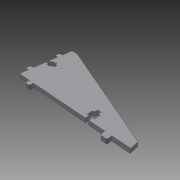
# Autodesk Inventor part: wiring_brace
Saved by Autodesk Inventor 2014 (Build 180170000, 170)
## iProperties
Created: 2013-12-07
Part Number: wiring_brace
Material: Generic
Document SubType Name: Modeling
Designer: buben
Density: 1 g/cm^3
Appearance: Default
Author: buben
Subject: Laser Cutted
Autodesk Inventor part; units mm, degrees
ref_plane "YZ Plane" through (0, 0, 0) normal (1, 0, 0) x (0, 1, 0)
ref_plane "XZ Plane" through (0, 0, 0) normal (0, 1, 0) x (-1, 0, 0)
ref_plane "XY Plane" through (0, 0, 0) normal (0, 0, 1) x (1, 0, 0)
sketch "Sketch1" plane through (0, 0, 0) normal (0, 0, 1) x (1, 0, 0)
  line L0 (0, 81) -> (0, 0)
  line L1 (0, 0) -> (161.5, 0)
  line L2 (161.5, 0) -> (161.5, 10)
  line L3 (161.5, 10) -> (10, 81)
  line L4 (10, 81) -> (0, 81)
  dimension "d0" = 161.5
  dimension "d1" = 81
  dimension "d2" = 10
  dimension "d3" = 10
  constraints: 10 end point, 2 parallel, 1 perpendicular, 1 vertical
  measures "d0" distance of L0.end L1.end
  measures "d1" distance of L0.start L0.end
  measures "d2" distance of L3.end L0.start
  measures "d3" distance of L1.end L2.end
extrude "Extrusion1" add sketch "Sketch1" along normal blind 6
sketch "Sketch2" plane through (0, 0, 6) normal (0, 0, 1) x (1, 0, 0)
  line L0 (0, 81) -> (0, 0) projected
  line L1 (0, 0) -> (161.5, 0) projected
  line L2 (161.5, 0) -> (161.5, 10) projected
  line L3 (16.3, 42.75) -> (16.3, 38.25)
  line L4 (0, 38.25) -> (0, 42.75)
  line L5 (5, 45.25) -> (12.3, 45.25)
  line L6 (12.3, 35.75) -> (5, 35.75)
  line L7 (0, 42.75) -> (5, 42.75)
  line L8 (12.3, 42.75) -> (16.3, 42.75)
  line L9 (16.3, 38.25) -> (12.3, 38.25)
  line L10 (5, 38.25) -> (0, 38.25)
  line L11 (5, 35.75) -> (5, 38.25)
  line L12 (5, 42.75) -> (5, 45.25)
  line L13 (12.3, 45.25) -> (12.3, 42.75)
  line L14 (12.3, 38.25) -> (12.3, 35.75)
  line L15 (109.25, 16.3) -> (113.75, 16.3)
  line L16 (113.75, 0) -> (109.25, 0)
  line L17 (116.25, 12.3) -> (116.25, 5)
  line L18 (106.75, 5) -> (106.75, 12.3)
  line L19 (106.75, 12.3) -> (109.25, 12.3)
  line L20 (113.75, 12.3) -> (116.25, 12.3)
  line L21 (116.25, 5) -> (113.75, 5)
  line L22 (109.25, 5) -> (106.75, 5)
  line L23 (109.25, 0) -> (109.25, 5)
  line L24 (109.25, 12.3) -> (109.25, 16.3)
  line L25 (113.75, 16.3) -> (113.75, 12.3)
  line L26 (113.75, 5) -> (113.75, 0)
  point P0 (16.3, 40.5)
  point P1 (0, 40.5)
  point P2 (111.5, 16.3)
  dimension "d6" = 4.5
  dimension "d7" = 2.5
  dimension "d8" = 2.5
  dimension "d9" = 5
  dimension "d10" = 7.3
  dimension "d11" = 4
  dimension "d12" = 4.5
  dimension "d13" = 5
  dimension "d14" = 7.3
  dimension "d15" = 4
  dimension "d16" = 2.5
  dimension "d17" = 2.5
  dimension "d18" = 50
  constraints: 48 end point, 20 parallel, 10 collinear, 8 perpendicular, 6 horizontal, 3 midpoint, 1 horizontal alignment
  measures "d6" distance of L3.start L3.end
  measures "d7" distance of L5.end L8.start
  measures "d8" distance of L9.end L6.start
  measures "d9" distance of L10.start L4.start
  measures "d10" distance of L6.start L6.end
  measures "d11" distance of L3.end L9.end
  measures "d12" distance of L15.start L15.end
  measures "d13" distance of L16.end L22.start
  measures "d14" distance of L18.start L18.end
  measures "d15" distance of L19.end L15.start
  measures "d16" distance of L18.end L19.end
  measures "d17" distance of L20.start L17.start
  measures "d18" distance from line of L2 point (111.5, 16.3)
extrude "Extrusion2" cut sketch "Sketch2" against normal blind 6
sketch "Sketch3" plane through (0, 0, 6) normal (0, 0, 1) x (1, 0, 0)
  line L0 (0, 38.25) -> (0, 0) projected
  line L1 (0, 0) -> (109.25, 0) projected
  line L2 (113.75, 0) -> (161.5, 0) projected
  line L3 (10, 81) -> (0, 81) projected
  line L4 (0, 81) -> (0, 42.75) projected
  line L5 (0, 65) -> (-4, 65)
  line L6 (-6, 63) -> (-6, 59)
  line L7 (-4, 57) -> (0, 57)
  line L8 (0, 57) -> (0, 65)
  line L9 (0, 20) -> (-4, 20)
  line L10 (-6, 18) -> (-6, 14)
  line L11 (-4, 12) -> (0, 12)
  line L12 (0, 12) -> (0, 20)
  line L13 (20, 0) -> (28, 0)
  line L14 (28, 0) -> (28, -4)
  line L15 (26, -6) -> (22, -6)
  line L16 (20, -4) -> (20, 0)
  line L17 (133.5, 0) -> (141.5, 0)
  line L18 (141.5, 0) -> (141.5, -4)
  line L19 (139.5, -6) -> (135.5, -6)
  line L20 (133.5, -4) -> (133.5, 0)
  arc A0 (-4, 65) -> (-6, 63) centre (-4, 63) ccw
  arc A1 (-6, 59) -> (-4, 57) centre (-4, 59) ccw
  arc A2 (-4, 20) -> (-6, 18) centre (-4, 18) ccw
  arc A3 (-6, 14) -> (-4, 12) centre (-4, 14) ccw
  arc A4 (20, -4) -> (22, -6) centre (22, -4) ccw
  arc A5 (26, -6) -> (28, -4) centre (26, -4) ccw
  arc A6 (133.5, -4) -> (135.5, -6) centre (135.5, -4) ccw
  arc A7 (139.5, -6) -> (141.5, -4) centre (139.5, -4) ccw
  dimension "d21" = 2
  dimension "d22" = 8
  dimension "d23" = 8
  dimension "d24" = 8
  dimension "d25" = 8
  dimension "d26" = 6
  dimension "d27" = 6
  dimension "d28" = 12
  dimension "d29" = 16
  dimension "d30" = 20
  dimension "d31" = 20
  constraints: 32 end point, 16 point on circle, 16 tangent, 8 centre point, 8 parallel, 7 equal radius, 4 horizontal, 4 perpendicular, 4 point on line, 2 collinear
  measures "d21" radius of A0
  measures "d22" distance between parallel lines of L7 L5
  measures "d23" distance between parallel lines of L11 L9
  measures "d24" distance between parallel lines of L14 L16
  measures "d25" distance between parallel lines of L18 L20
  measures "d26" distance between parallel lines of L8 L6
  measures "d27" distance between parallel lines of L1 L15
  measures "d28" distance between parallel lines of L1 L11
  measures "d29" distance between parallel lines of L3 L5
  measures "d30" distance between parallel lines of L0 L16
  measures "d31" distance from line of L2.end L18
extrude "Extrusion3" add sketch "Sketch3" against normal blind 6
body "Solid1"
